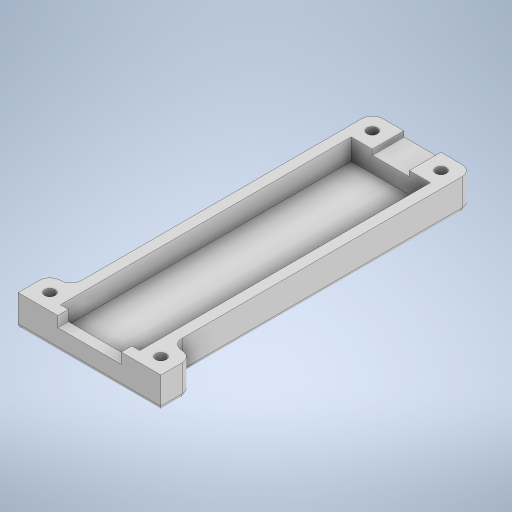
# Autodesk Inventor part: Case Bawah
Saved by Autodesk Inventor 2024 (Build 280153000, 153)
## iProperties
Created: 2023-08-08
Part Number: Case Bawah
Material: Generic
Document SubType Name: Modeling
Designer: Asus
Density: 1 g/cm^3
Appearance: Default
Author: Asus
## iProperties of the stored document Case Bawah_3DPrint.ipt
Created: 2023-08-08
Part Number: Case Bawah_3DPrint
Material: Generic
Document SubType Name: Modeling
Designer: Asus
Density: 1 g/cm^3
Appearance: Default
Author: Asus
Autodesk Inventor part; units mm, degrees
ref_plane "YZ Plane" through (0, 0, 0) normal (1, 0, 0) x (0, 1, 0)
ref_plane "XZ Plane" through (0, 0, 0) normal (0, 1, 0) x (-1, 0, 0)
ref_plane "XY Plane" through (0, 0, 0) normal (0, 0, 1) x (1, 0, 0)
sketch "Sketch2" plane through (0, 0, 0) normal (0, 1, 0) x (-1, 0, 0)
  line L0 (0, 0) -> (0, -2)
  line L1 (0, -2) -> (2, -2) construction
  line L2 (2, -2) -> (17, -2) construction
  line L3 (17, -2) -> (17, -57) construction
  line L4 (2, -2) -> (17, -2)
  line L5 (17, -2) -> (17, -57)
  line L6 (17, -57) -> (2, -57)
  line L7 (2, -57) -> (2, -2)
  line L8 (17, -57) -> (17, -63) construction
  line L9 (17, -63) -> (19, -63) construction
  line L10 (0, 0) -> (19, 0)
  line L11 (19, -8) -> (19, -63)
  line L12 (19, -63) -> (0, -63)
  line L13 (0, -63) -> (0, -8)
  line L14 (19, 0) -> (23, 0)
  line L15 (23, 0) -> (23, -4)
  line L16 (21, -6) -> (21, -6)
  arc A0 (21, -6) -> (19, -8) centre (21, -8) ccw
  arc A1 (21, -6) -> (23, -4) centre (21, -4) ccw
  line L17 (0, 0) -> (-4, 0)
  line L18 (-4, 0) -> (-4, -4)
  line L19 (-2, -6) -> (-2, -6)
  arc A2 (0, -8) -> (-2, -6) centre (-2, -8) ccw
  arc A3 (-4, -4) -> (-2, -6) centre (-2, -4) ccw
  line L20 (23, 0) -> (23, -3) construction
  line L21 (0, 0) -> (-1, 0) construction
  line L22 (-1, 0) -> (-1, -3) construction
  circle A4 centre (-1, -3) radius 1
  line L23 (23, 0) -> (23, -3) construction
  line L24 (23, -3) -> (20, -3) construction
  line L25 (20, -3) -> (22, -3) construction
  circle A5 centre (20, -3) radius 1
  line L26 (22, -4.1547) -> (20, -5.3094)
  line L27 (20, -5.3094) -> (18, -4.1547)
  line L28 (18, -4.1547) -> (18, -1.8453)
  line L29 (18, -1.8453) -> (20, -0.6906)
  line L30 (20, -0.6906) -> (22, -1.8453)
  line L31 (22, -1.8453) -> (22, -4.1547)
  line L32 (-1, -3) -> (1, -3) construction
  line L33 (1, -4.1547) -> (-1, -5.3094)
  line L34 (-1, -5.3094) -> (-3, -4.1547)
  line L35 (-3, -4.1547) -> (-3, -1.8453)
  line L36 (-3, -1.8453) -> (-1, -0.6906)
  line L37 (-1, -0.6906) -> (1, -1.8453)
  line L38 (1, -1.8453) -> (1, -4.1547)
  line L39 (0, -63) -> (0, -60) construction
  line L40 (0, -60) -> (3, -60) construction
  line L41 (19, -63) -> (19, -60) construction
  line L42 (19, -60) -> (16, -60) construction
  line L43 (16, -60) -> (14, -60) construction
  line L44 (3, -60) -> (5, -60) construction
  circle A6 centre (3, -60) radius 1
  circle A7 centre (16, -60) radius 1
  line L45 (5, -61.1547) -> (3, -62.3094)
  line L46 (3, -62.3094) -> (1, -61.1547)
  line L47 (1, -61.1547) -> (1, -58.8453)
  line L48 (1, -58.8453) -> (3, -57.6906)
  line L49 (3, -57.6906) -> (5, -58.8453)
  line L50 (5, -58.8453) -> (5, -61.1547)
  line L51 (14, -58.8453) -> (16, -57.6906)
  line L52 (16, -57.6906) -> (18, -58.8453)
  line L53 (18, -58.8453) -> (18, -61.1547)
  line L54 (18, -61.1547) -> (16, -62.3094)
  line L55 (16, -62.3094) -> (14, -61.1547)
  line L56 (14, -61.1547) -> (14, -58.8453)
  point P0 (23, -6)
  point P1 (-4, -6)
  dimension "d4" = 2
  dimension "d5" = 2
  dimension "d6" = 15
  dimension "d8" = 6
  dimension "d9" = 2
  dimension "d15" = 4
  dimension "d16" = 6
  dimension "d17" = 2
  dimension "d18" = 4
  dimension "d19" = 6
  dimension "d20" = 2
  dimension "d34" = 1
  dimension "d35" = 3
  dimension "d36" = 2
  dimension "d39" = 3
  dimension "d40" = 3
  dimension "d41" = 2
  dimension "d42" = 2
  dimension "d43" = 2
  dimension "d52" = 3
  dimension "d53" = 3
  dimension "d54" = 3
  dimension "d55" = 3
  dimension "d56" = 2
  dimension "d57" = 2
  dimension "d58" = 2
  dimension "d59" = 2
  constraints: 114 end point, 15 point on line, 13 perpendicular, 8 centre point, 8 coincident, 8 point on circle, 8 tangent, 5 horizontal, 4 midpoint, 4 parallel, 2 equal radius, 2 vertical, 52 other
  measures "d4" distance of L0.start L0.end
  measures "d5" distance of L0.end L1.end
  measures "d6" distance of L1.end L2.end
  measures "d8" distance of L3.end L8.end
  measures "d9" distance of L8.end L9.end
  measures "d15" distance of L10.end L14.end
  measures "d16" distance of L14.end point (23, -6)
  measures "d17" radius of A0
  measures "d18" distance of L0.start L17.end
  measures "d19" distance of L17.end point (-4, -6)
  measures "d20" radius of A2
  measures "d34" distance of L0.start L21.end
  measures "d35" distance of L21.end L22.end
  measures "d36" diameter of A4
  measures "d39" distance of L14.end L20.end
  measures "d40" distance of L20.end L24.end
  measures "d41" distance of L24.end L25.end
  measures "d42" diameter of A5
  measures "d43" distance of L32.start L32.end
  measures "d52" distance of L12.end L39.end
  measures "d53" distance of L39.end L40.end
  measures "d54" distance of L9.end L41.end
  measures "d55" distance of L41.end L42.end
  measures "d56" distance of L42.end L43.end
  measures "d57" distance of L40.end L44.end
  measures "d58" diameter of A6
  measures "d59" diameter of A7
extrude "Extrusion7" add sketch "Sketch2" along normal blind 6 contours L10 L14 L15 A1 A0 L11 L12 L13 A2 A3 L18 L17 | L26 L27 L28 L29 L30 L31 | L33 L34 L35 L36 L37 L38 | L45 L46 L47 L48 L49 L50 | L51 L52 L53 L54 L55 L56
extrude "Extrusion8" cut sketch "Sketch2" along normal blind 2 contours L26 L27 L28 L29 L30 L31 | L33 L34 L35 L36 L37 L38 | L45 L46 L47 L48 L49 L50 | L51 L52 L53 L54 L55 L56
extrude "Extrusion9" add sketch "Sketch2" along normal blind 2 contours L4 L5 L6 L7
sketch "Sketch7" plane through (-23, 0, 0) normal (0, 0, 1) x (1, 0, 0)
  line L0 (0, 0) -> (0, 6) construction
  line L1 (0, 6) -> (27, 6) construction
  line L2 (0, 6) -> (27, 6) construction
  line L3 (13.5, 6) -> (13.5, 4) construction
  line L4 (13.5, 4) -> (19.5, 4) construction
  line L5 (19.5, 4) -> (7.5, 4)
  line L6 (7.5, 4) -> (7.5, 6)
  line L7 (7.5, 6) -> (19.5, 6)
  line L8 (19.5, 6) -> (19.5, 4)
  point P0 (23, 0)
  dimension "d62" = 2
  dimension "d63" = 6
  dimension "d64" = 12
  constraints: 14 end point, 3 parallel, 1 collinear, 1 horizontal, 1 midpoint, 1 perpendicular, 1 point on line, 1 vertical
  measures "d62" distance of L3.start L3.end
  measures "d63" distance of L3.end L4.end
  measures "d64" distance of L6.end L7.end
extrude "Extrusion10" cut sketch "Sketch7" against normal blind 2
sketch "Sketch9" plane through (0, 0, -63) normal (0, 0, -1) x (-1, 0, 0)
  line L0 (0, 0) -> (0, 6) construction
  line L1 (0, 6) -> (19, 6) construction
  line L2 (0, 6) -> (19, 6) construction
  line L3 (9.5, 6) -> (9.5, 5) construction
  line L4 (9.5, 5) -> (13, 5) construction
  line L5 (13, 5) -> (6, 5)
  line L6 (6, 5) -> (6, 6)
  line L7 (6, 6) -> (13, 6)
  line L8 (13, 6) -> (13, 5)
  dimension "d67" = 1
  dimension "d68" = 3.5
  dimension "d69" = 7
  constraints: 14 end point, 3 equal length, 2 perpendicular, 1 horizontal, 1 midpoint, 1 point on line, 1 vertical
  measures "d67" distance of L3.start L3.end
  measures "d68" distance of L3.end L4.end
  measures "d69" distance of L6.end L7.end
extrude "Extrusion11" cut sketch "Sketch9" against normal blind 6
fillet "Fillet1" radius 2 2 edges at (0, 3, -63) (-19, 3, -63)
fillet "Fillet2" radius 0.9 12 edges at (-22.4142, 0, -5.4142) (-23, 0, -2) (-19, 0, -34.5) (-18.4142, 0, -62.4142) (-9.5, 0, -63) (-0.5858, 0, -62.4142) (0, 0, -34.5) (0.5858, 0, -6.5858) (3.4142, 0, -5.4142) (4, 0, -2) (-19.5858, 0, -6.5858) (-9.5, 0, 0)
body "Solid6"
